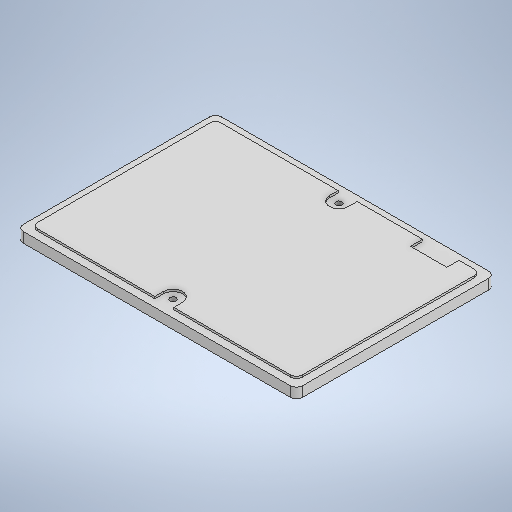
# Autodesk Inventor part: Lid
Saved by Autodesk Inventor 2025 (Build 290162000, 162)
## iProperties
Created: 2024-06-09
Part Number: Lid
Material: Generic
Document SubType Name: Modeling
Designer: Dell
Density: 1 g/cm^3
Appearance: Default
Author: Dell
Autodesk Inventor part; units mm, degrees
ref_plane "YZ Plane" through (0, 0, 0) normal (1, 0, 0) x (0, 1, 0)
ref_plane "XZ Plane" through (0, 0, 0) normal (0, 1, 0) x (-1, 0, 0)
ref_plane "XY Plane" through (0, 0, 0) normal (0, 0, 1) x (1, 0, 0)
sketch "Sketch1" plane through (0, 0, 0) normal (0, 1, 0) x (-1, 0, 0)
  line L0 (59, 49.2) -> (-66, 49.2)
  arc A0 (-66, 49.2) -> (-69, 46.2) centre (-66, 46.2) ccw
  line L1 (-69, 46.2) -> (-69, -38.8)
  arc A1 (-69, -38.8) -> (-66, -41.8) centre (-66, -38.8) ccw
  line L2 (-66, -41.8) -> (59, -41.8)
  arc A2 (59, -41.8) -> (62, -38.8) centre (59, -38.8) ccw
  line L3 (62, -38.8) -> (62, 46.2)
  arc A3 (62, 46.2) -> (59, 49.2) centre (59, 46.2) ccw
  line L4 (65.5, 49.7) -> (65.5, -42.3)
  line L5 (62.5, -45.3) -> (-69.5, -45.3)
  line L6 (-72.5, -42.3) -> (-72.5, 49.7)
  line L7 (-69.5, 52.7) -> (62.5, 52.7)
  arc A4 (62.5, -45.3) -> (65.5, -42.3) centre (62.5, -42.3) ccw
  arc A5 (-72.5, -42.3) -> (-69.5, -45.3) centre (-69.5, -42.3) ccw
  arc A6 (-69.5, 52.7) -> (-72.5, 49.7) centre (-69.5, 49.7) ccw
  arc A7 (65.5, 49.7) -> (62.5, 52.7) centre (62.5, 49.7) ccw
  point P0 (65.5, -38.8)
  point P1 (59, -45.3)
  dimension "d0" = 3
  dimension "d3" = 131
  dimension "d6" = 91
  dimension "d29" = 3.5
  dimension "d44" = 3
  dimension "d45" = 3
  dimension "d46" = 3
  dimension "d47" = 3
  constraints: 16 end point, 16 point on circle, 16 tangent, 8 centre point, 4 parallel, 3 equal radius, 2 point on line, 1 horizontal, 1 vertical
  measures "d0" radius of A3
  measures "d3" distance between parallel lines of L3 L1
  measures "d6" distance between parallel lines of L0 L2
  measures "d29" distance between parallel lines of L3 L4
  measures "d44" radius of A4
  measures "d45" radius of A5
  measures "d46" radius of A6
  measures "d47" radius of A7
extrude "Extrusion6" add sketch "Sketch1" along normal blind 1.5 contours A3 L3 A2 L2 A1 L1 A0 L0
extrude "Extrusion7" add sketch "Sketch1" along normal blind 5
sketch "Sketch3" plane through (0, 1.5, 0) normal (0, 1, 0) x (1, 0, 0)
  line L0 (-59, 41.8) -> (66, 41.8) projected
  line L1 (66, -49.2) -> (-59, -49.2) projected
  circle A0 centre (3.5, 37.3) radius 1.5
  circle A1 centre (3.5, 37.3) radius 4.5
  line L2 (8, 37.3) -> (8, 41.8)
  line L3 (-1, 37.3) -> (-1, 41.8)
  line L4 (-62, 38.8) -> (-62, -46.2) projected
  line L5 (-62, -3.7) -> (-24.2248, -3.7)
  circle A2 centre (3.5, -44.7) radius 1.5
  circle A3 centre (3.5, -44.7) radius 4.5
  line L6 (8, -44.7) -> (8, -49.2)
  line L7 (-1, -44.7) -> (-1, -49.2)
  point P0 (0, 0)
  dimension "d34" = 3
  dimension "d35" = 9
  dimension "d36" = 4.5
  constraints: 10 end point, 6 symmetric about line, 4 centre point, 4 point on circle, 2 coincident, 2 perpendicular, 2 point on line, 2 tangent, 1 horizontal, 1 midpoint, 2 other
  measures "d34" diameter of A0
  measures "d35" diameter of A1
  measures "d36" distance from line of L0 A0.centre
extrude "Extrusion8" add sketch "Sketch3" along normal blind 3.5
sketch "Sketch4" plane through (0, 1.5, 0) normal (0, 1, 0) x (1, 0, 0)
  line L0 (8, 41.8) -> (8, 37.3) projected
  arc A0 (-1, 37.3) -> (8, 37.3) centre (3.5, 37.3) ccw projected
  line L1 (-1, 37.3) -> (-1, 41.8) projected
  line L2 (-1, 41.8) -> (-59, 41.8) projected
  arc A1 (-59, 41.8) -> (-62, 38.8) centre (-59, 38.8) ccw projected
  line L3 (-62, 38.8) -> (-62, -46.2) projected
  arc A2 (-62, -46.2) -> (-59, -49.2) centre (-59, -46.2) ccw projected
  line L4 (-59, -49.2) -> (-1, -49.2) projected
  line L5 (-1, -49.2) -> (-1, -44.7) projected
  arc A3 (8, -44.7) -> (-1, -44.7) centre (3.5, -44.7) ccw projected
  line L6 (8, -44.7) -> (8, -49.2) projected
  line L7 (8, -49.2) -> (66, -49.2) projected
  arc A4 (66, -49.2) -> (69, -46.2) centre (66, -46.2) ccw projected
  line L8 (69, -46.2) -> (69, 38.8) projected
  arc A5 (69, 38.8) -> (66, 41.8) centre (66, 38.8) ccw projected
  line L9 (66, 41.8) -> (8, 41.8) projected
  line L10 (-59, 41.6) -> (-1.2, 41.6)
  line L11 (-1.2, 41.6) -> (-1.2, 37.3)
  arc A6 (-1.2, 37.3) -> (8.2, 37.3) centre (3.5, 37.3) ccw
  line L12 (8.2, 37.3) -> (8.2, 41.6)
  line L13 (8.2, 41.6) -> (66, 41.6)
  arc A7 (68.8, 38.8) -> (66, 41.6) centre (66, 38.8) ccw
  line L14 (68.8, 38.8) -> (68.8, -46.2)
  arc A8 (66, -49) -> (68.8, -46.2) centre (66, -46.2) ccw
  line L15 (66, -49) -> (8.2, -49)
  line L16 (8.2, -49) -> (8.2, -44.7)
  arc A9 (8.2, -44.7) -> (-1.2, -44.7) centre (3.5, -44.7) ccw
  line L17 (-1.2, -44.7) -> (-1.2, -49)
  line L18 (-1.2, -49) -> (-59, -49)
  arc A10 (-61.8, -46.2) -> (-59, -49) centre (-59, -46.2) ccw
  line L19 (-61.8, -46.2) -> (-61.8, 38.8)
  arc A11 (-59, 41.6) -> (-61.8, 38.8) centre (-59, 38.8) ccw
  point P0 (0, 0)
  dimension "d39" = 0.2
  constraints: 20 end point, 12 point on circle, 6 centre point, 15 other
  measures "d39" distance between parallel lines of L2 L10
extrude "Extrusion9" add sketch "Sketch4" along normal blind 3.5
extrude "Extrusion10" add sketch "Sketch4" along normal blind 4.5 contours L10 L11 A6 L12 L13 A7 L14 A8 L15 L16 A9 L17 L18 A10 L19 A11
sketch "Sketch5" plane through (0, 6, 0) normal (0, 1, 0) x (1, 0, 0)
  line L0 (66, 41.6) -> (8.2, 41.6) projected
  line L1 (40.5, 41.6) -> (58.5, 41.6)
  line L2 (58.5, 41.6) -> (58.5, 35.6)
  line L3 (58.5, 35.6) -> (40.5, 35.6)
  line L4 (40.5, 35.6) -> (40.5, 41.6)
  point P0 (0, 0)
  point P1 (69.5, 45.3)
  point P2 (49.5, 41.6)
  dimension "d48" = 18
  dimension "d49" = 6
  dimension "d50" = 20
  constraints: 8 end point, 2 parallel, 1 horizontal, 1 midpoint, 1 perpendicular, 1 point on line
  measures "d48" distance of L2.end L3.end
  measures "d49" distance of L1.end L2.end
  measures "d50" horizontal distance of point (49.5, 41.6) point (69.5, 45.3)
extrude "Extrusion11" cut sketch "Sketch5" against normal up to surface (1 mm away)
sketch "Sketch6" plane through (0, 0, 0) normal (0, -1, 0) x (1, 0, 0)
  circle A0 centre (3.5, -37.3) radius 1.5 projected
  arc A1 (8.2, -37.3) -> (-1.2, -37.3) centre (3.5, -37.3) ccw projected
  circle A2 centre (3.5, 44.7) radius 1.5 projected
  arc A3 (-1.2, 44.7) -> (8.2, 44.7) centre (3.5, 44.7) ccw projected
  circle A4 centre (3.5, -37.3) radius 2.75
  circle A5 centre (3.5, 44.7) radius 2.75
  point P0 (0, 0)
  dimension "d55" = 5.5
  dimension "d56" = 5.5
  constraints: 2 centre point, 2 coincident
  measures "d55" diameter of A4
  measures "d56" diameter of A5
extrude "Extrusion12" cut sketch "Sketch6" against normal blind 10 contours A0 | A2
extrude "Extrusion13" cut sketch "Sketch6" against normal blind 2
sketch "Sketch7" plane through (0, 0, 0) normal (0, -1, 0) x (1, 0, 0)
  line L0 (-65.5, -42.3) -> (-65.5, 49.7) projected
  line L1 (-62.5, 52.7) -> (69.5, 52.7) projected
  line L2 (72.5, 49.7) -> (72.5, -42.3) projected
  line L3 (69.5, -45.3) -> (-62.5, -45.3) projected
  line L4 (-34.3067, 8.9219) -> (41.3173, 8.9219) construction
  line L5 (41.3173, 8.9219) -> (41.3173, -1.4995) construction
  line L6 (41.3173, -1.4995) -> (-34.3067, -1.4995) construction
  line L7 (-34.3067, -1.4995) -> (-34.3067, 8.9219) construction
  line L8 (-53.3099, -3.7888) -> (-48.2532, 11.2112)
  line L9 (-48.2532, 11.2112) -> (-45.7977, 11.2112)
  line L10 (-45.7977, 11.2112) -> (-40.741, -3.7888)
  line L11 (-40.741, -3.7888) -> (-42.8439, -3.7888)
  line L12 (-42.8439, -3.7888) -> (-44.2054, 0.4049)
  line L13 (-44.2054, 0.4049) -> (-49.9306, 0.4049)
  line L14 (-49.9306, 0.4049) -> (-51.2921, -3.7888)
  line L15 (-51.2921, -3.7888) -> (-53.3099, -3.7888)
  line L16 (-44.7524, 2.1067) -> (-47.0741, 9.1691)
  line L17 (-47.0741, 9.1691) -> (-49.3836, 2.1067)
  line L18 (-49.3836, 2.1067) -> (-44.7524, 2.1067)
  spline S0 degree 2 poles (-33.0344, -4.0805) (-34.6268, -4.0805) (-37.2645, -3.1081) (-38.2127, -2.1235) knots 0 0 0 1 2 2 2
  spline S1 degree 2 poles (-38.2127, -2.1235) (-39.1608, -1.1267) (-40.1697, 1.8149) (-40.1697, 3.7234) knots 0 0 0 1 2 2 2
  spline S2 degree 2 poles (-40.1697, 3.7234) (-40.1697, 5.5346) (-39.1486, 8.4033) (-38.2005, 9.4243) knots 0 0 0 1 2 2 2
  spline S3 degree 2 poles (-38.2005, 9.4243) (-37.2888, 10.4089) (-34.6146, 11.4786) (-33.0222, 11.4786) knots 0 0 0 1 2 2 2
  spline S4 degree 2 poles (-33.0222, 11.4786) (-32.2564, 11.4786) (-30.8707, 11.2598) (-30.2386, 11.0653) knots 0 0 0 1 2 2 2
  spline S5 degree 2 poles (-30.2386, 11.0653) (-29.7281, 10.9195) (-28.4882, 10.3846) (-28.1114, 10.1901) knots 0 0 0 1 2 2 2
  line L19 (-28.1114, 10.1901) -> (-28.1114, 7.7833)
  line L20 (-28.1114, 7.7833) -> (-28.2815, 7.7833)
  spline S6 degree 2 poles (-28.2815, 7.7833) (-28.6584, 8.1115) (-29.4485, 8.7072) (-30.1778, 9.0475) knots 0 0 0 1 2 2 2
  spline S7 degree 2 poles (-30.1778, 9.0475) (-30.7856, 9.3514) (-32.3537, 9.7525) (-33.2532, 9.7525) knots 0 0 0 1 2 2 2
  spline S8 degree 2 poles (-33.2532, 9.7525) (-35.4169, 9.7525) (-38.0911, 6.4948) (-38.0911, 3.7841) knots 0 0 0 1 2 2 2
  spline S9 degree 2 poles (-38.0911, 3.7841) (-38.0911, 2.2769) (-37.3861, 0.0159) (-36.7175, -0.762) knots 0 0 0 1 2 2 2
  spline S10 degree 2 poles (-36.7175, -0.762) (-36.0733, -1.54) (-34.2499, -2.3544) (-33.1073, -2.3544) knots 0 0 0 1 2 2 2
  spline S11 degree 2 poles (-33.1073, -2.3544) (-32.2686, -2.3544) (-30.5911, -2.1113) (-30.0198, -1.8682) knots 0 0 0 1 2 2 2
  line L21 (-30.0198, -1.8682) -> (-30.0198, 2.0094)
  line L22 (-30.0198, 2.0094) -> (-33.4963, 2.0094)
  line L23 (-33.4963, 2.0094) -> (-33.4963, 3.7598)
  line L24 (-33.4963, 3.7598) -> (-28.0506, 3.7598)
  line L25 (-28.0506, 3.7598) -> (-28.0506, -2.792)
  spline S12 degree 2 poles (-28.0506, -2.792) (-28.4274, -2.9622) (-29.7159, -3.4849) (-30.2629, -3.6429) knots 0 0 0 1 2 2 2
  spline S13 degree 2 poles (-30.2629, -3.6429) (-31.0044, -3.8617) (-32.1956, -4.0805) (-33.0344, -4.0805) knots 0 0 0 1 2 2 2
  line L26 (-13.9379, -3.7888) -> (-16.5271, -3.7888)
  line L27 (-16.5271, -3.7888) -> (-21.2678, 2.1796)
  line L28 (-21.2678, 2.1796) -> (-23.553, 2.1796)
  line L29 (-23.553, 2.1796) -> (-23.553, -3.7888)
  line L30 (-23.553, -3.7888) -> (-25.5465, -3.7888)
  line L31 (-25.5465, -3.7888) -> (-25.5465, 11.2112)
  line L32 (-25.5465, 11.2112) -> (-21.681, 11.2112)
  spline S14 degree 2 poles (-21.681, 11.2112) (-20.3926, 11.2112) (-18.6543, 10.9316) (-17.8642, 10.4211) knots 0 0 0 1 2 2 2
  spline S15 degree 2 poles (-17.8642, 10.4211) (-17.0741, 9.9106) (-16.1624, 8.3182) (-16.1624, 7.1391) knots 0 0 0 1 2 2 2
  spline S16 degree 2 poles (-16.1624, 7.1391) (-16.1624, 5.4981) (-17.8399, 3.2736) (-19.2742, 2.7388) knots 0 0 0 1 2 2 2
  line L33 (-19.2742, 2.7388) -> (-13.9379, -3.7888)
  spline S17 degree 2 poles (-18.241, 6.9811) (-18.241, 7.6375) (-18.7029, 8.6464) (-19.1892, 8.9746) knots 0 0 0 1 2 2 2
  spline S18 degree 2 poles (-19.1892, 8.9746) (-19.6146, 9.2542) (-20.7451, 9.4851) (-21.5716, 9.4851) knots 0 0 0 1 2 2 2
  line L34 (-21.5716, 9.4851) -> (-23.553, 9.4851)
  line L35 (-23.553, 9.4851) -> (-23.553, 3.8449)
  line L36 (-23.553, 3.8449) -> (-21.8026, 3.8449)
  spline S19 degree 2 poles (-21.8026, 3.8449) (-20.9396, 3.8449) (-19.566, 4.1488) (-19.0919, 4.6229) knots 0 0 0 1 2 2 2
  spline S20 degree 2 poles (-19.0919, 4.6229) (-18.6543, 5.0362) (-18.241, 6.2031) (-18.241, 6.9811) knots 0 0 0 1 2 2 2
  spline S21 degree 2 poles (-2.1349, 9.4973) (-1.284, 8.5005) (-0.3358, 5.5832) (-0.3358, 3.7112) knots 0 0 0 1 2 2 2
  spline S22 degree 2 poles (-0.3358, 3.7112) (-0.3358, 1.8879) (-1.2597, -1.0659) (-2.1349, -2.0627) knots 0 0 0 1 2 2 2
  spline S23 degree 2 poles (-2.1349, -2.0627) (-3.0587, -3.1081) (-5.502, -4.1048) (-6.9728, -4.1048) knots 0 0 0 1 2 2 2
  spline S24 degree 2 poles (-6.9728, -4.1048) (-8.4922, -4.1048) (-10.9234, -3.0716) (-11.8107, -2.0627) knots 0 0 0 1 2 2 2
  spline S25 degree 2 poles (-11.8107, -2.0627) (-12.6738, -1.0659) (-13.5976, 1.8636) (-13.5976, 3.7112) knots 0 0 0 1 2 2 2
  spline S26 degree 2 poles (-13.5976, 3.7112) (-13.5976, 5.5953) (-12.6616, 8.4641) (-11.7986, 9.4973) knots 0 0 0 1 2 2 2
  spline S27 degree 2 poles (-11.7986, 9.4973) (-10.9234, 10.494) (-8.4801, 11.5273) (-6.9728, 11.5273) knots 0 0 0 1 2 2 2
  spline S28 degree 2 poles (-6.9728, 11.5273) (-5.4412, 11.5273) (-2.9857, 10.4576) (-2.1349, 9.4973) knots 0 0 0 1 2 2 2
  spline S29 degree 2 poles (-2.4144, 3.7112) (-2.4144, 5.1942) (-3.0587, 7.4916) (-3.6422, 8.2452) knots 0 0 0 1 2 2 2
  spline S30 degree 2 poles (-3.6422, 8.2452) (-4.2378, 9.0232) (-5.9152, 9.8012) (-6.9606, 9.8012) knots 0 0 0 1 2 2 2
  spline S31 degree 2 poles (-6.9606, 9.8012) (-8.0425, 9.8012) (-9.6713, 9.0475) (-10.2913, 8.2452) knots 0 0 0 1 2 2 2
  spline S32 degree 2 poles (-10.2913, 8.2452) (-10.8869, 7.4794) (-11.519, 5.1699) (-11.519, 3.7112) knots 0 0 0 1 2 2 2
  spline S33 degree 2 poles (-11.519, 3.7112) (-11.519, 0.7574) (-9.0392, -2.3787) (-6.9606, -2.3787) knots 0 0 0 1 2 2 2
  spline S34 degree 2 poles (-6.9606, -2.3787) (-4.882, -2.3787) (-2.4144, 0.7574) (-2.4144, 3.7112) knots 0 0 0 1 2 2 2
  spline S35 degree 2 poles (6.0337, -4.0562) (4.4049, -4.0562) (2.1196, -3.3755) (1.1107, -2.8893) knots 0 0 0 1 2 2 2
  line L37 (1.1107, -2.8893) -> (1.1107, -0.3852)
  line L38 (1.1107, -0.3852) -> (1.2566, -0.3852)
  spline S36 degree 2 poles (1.2566, -0.3852) (2.2412, -1.309) (4.7331, -2.3301) (5.8878, -2.3301) knots 0 0 0 1 2 2 2
  spline S37 degree 2 poles (5.8878, -2.3301) (7.541, -2.3301) (9.2306, -0.9565) (9.2306, 0.1739) knots 0 0 0 1 2 2 2
  spline S38 degree 2 poles (9.2306, 0.1739) (9.2306, 1.0735) (8.3433, 2.1918) (7.383, 2.4713) knots 0 0 0 1 2 2 2
  spline S39 degree 2 poles (7.383, 2.4713) (6.6901, 2.6658) (5.5353, 2.9333) (4.6723, 3.1521) knots 0 0 0 1 2 2 2
  spline S40 degree 2 poles (4.6723, 3.1521) (3.8943, 3.3587) (2.6666, 3.9786) (2.1925, 4.477) knots 0 0 0 1 2 2 2
  spline S41 degree 2 poles (2.1925, 4.477) (1.7306, 4.9754) (1.2201, 6.3125) (1.2201, 7.1877) knots 0 0 0 1 2 2 2
  spline S42 degree 2 poles (1.2201, 7.1877) (1.2201, 9.0111) (4.0645, 11.4786) (6.2647, 11.4786) knots 0 0 0 1 2 2 2
  spline S43 degree 2 poles (6.2647, 11.4786) (7.5288, 11.4786) (9.7655, 10.9803) (10.7258, 10.5062) knots 0 0 0 1 2 2 2
  line L39 (10.7258, 10.5062) -> (10.7258, 8.1237)
  line L40 (10.7258, 8.1237) -> (10.5799, 8.1237)
  spline S44 degree 2 poles (10.5799, 8.1237) (9.8627, 8.7801) (7.6261, 9.7525) (6.3984, 9.7525) knots 0 0 0 1 2 2 2
  spline S45 degree 2 poles (6.3984, 9.7525) (5.0126, 9.7525) (3.2987, 8.4519) (3.2987, 7.3944) knots 0 0 0 1 2 2 2
  spline S46 degree 2 poles (3.2987, 7.3944) (3.2987, 6.4462) (4.3076, 5.3158) (5.2557, 5.0605) knots 0 0 0 1 2 2 2
  spline S47 degree 2 poles (5.2557, 5.0605) (5.8878, 4.8903) (7.7233, 4.4527) (8.3311, 4.2704) knots 0 0 0 1 2 2 2
  spline S48 degree 2 poles (8.3311, 4.2704) (9.8749, 3.7963) (11.3092, 1.8879) (11.3092, 0.49) knots 0 0 0 1 2 2 2
  spline S49 degree 2 poles (11.3092, 0.49) (11.3092, -0.3974) (10.592, -2.0992) (9.9478, -2.6948) knots 0 0 0 1 2 2 2
  spline S50 degree 2 poles (9.9478, -2.6948) (9.2306, -3.3512) (7.4073, -4.0562) (6.0337, -4.0562) knots 0 0 0 1 2 2 2
  line L41 (13.3392, -3.7888) -> (13.3392, 11.2112)
  line L42 (13.3392, 11.2112) -> (22.7233, 11.2112)
  line L43 (22.7233, 11.2112) -> (22.7233, 9.4365)
  line L44 (22.7233, 9.4365) -> (15.3327, 9.4365)
  line L45 (15.3327, 9.4365) -> (15.3327, 5.3279)
  line L46 (15.3327, 5.3279) -> (22.2249, 5.3279)
  line L47 (22.2249, 5.3279) -> (22.2249, 3.5532)
  line L48 (22.2249, 3.5532) -> (15.3327, 3.5532)
  line L49 (15.3327, 3.5532) -> (15.3327, -2.0141)
  line L50 (15.3327, -2.0141) -> (22.7233, -2.0141)
  line L51 (22.7233, -2.0141) -> (22.7233, -3.7888)
  line L52 (22.7233, -3.7888) -> (13.3392, -3.7888)
  line L53 (35.6447, -3.7888) -> (33.4081, -3.7888)
  line L54 (33.4081, -3.7888) -> (26.7711, 9.1448)
  line L55 (26.7711, 9.1448) -> (26.7711, -3.7888)
  line L56 (26.7711, -3.7888) -> (24.9113, -3.7888)
  line L57 (24.9113, -3.7888) -> (24.9113, 11.2112)
  line L58 (24.9113, 11.2112) -> (27.7436, 11.2112)
  line L59 (27.7436, 11.2112) -> (33.7849, -0.6648)
  line L60 (33.7849, -0.6648) -> (33.7849, 11.2112)
  line L61 (33.7849, 11.2112) -> (35.6447, 11.2112)
  line L62 (35.6447, 11.2112) -> (35.6447, -3.7888)
  spline S51 degree 2 poles (42.8651, -4.0562) (41.2363, -4.0562) (38.951, -3.3755) (37.9421, -2.8893) knots 0 0 0 1 2 2 2
  line L63 (37.9421, -2.8893) -> (37.9421, -0.3852)
  line L64 (37.9421, -0.3852) -> (38.088, -0.3852)
  spline S52 degree 2 poles (38.088, -0.3852) (39.0726, -1.309) (41.5645, -2.3301) (42.7193, -2.3301) knots 0 0 0 1 2 2 2
  spline S53 degree 2 poles (42.7193, -2.3301) (44.3724, -2.3301) (46.0621, -0.9565) (46.0621, 0.1739) knots 0 0 0 1 2 2 2
  spline S54 degree 2 poles (46.0621, 0.1739) (46.0621, 1.0735) (45.1747, 2.1918) (44.2144, 2.4713) knots 0 0 0 1 2 2 2
  spline S55 degree 2 poles (44.2144, 2.4713) (43.5215, 2.6658) (42.3668, 2.9333) (41.5037, 3.1521) knots 0 0 0 1 2 2 2
  spline S56 degree 2 poles (41.5037, 3.1521) (40.7258, 3.3587) (39.498, 3.9786) (39.024, 4.477) knots 0 0 0 1 2 2 2
  spline S57 degree 2 poles (39.024, 4.477) (38.5621, 4.9754) (38.0515, 6.3125) (38.0515, 7.1877) knots 0 0 0 1 2 2 2
  spline S58 degree 2 poles (38.0515, 7.1877) (38.0515, 9.0111) (40.8959, 11.4786) (43.0961, 11.4786) knots 0 0 0 1 2 2 2
  spline S59 degree 2 poles (43.0961, 11.4786) (44.3603, 11.4786) (46.5969, 10.9803) (47.5572, 10.5062) knots 0 0 0 1 2 2 2
  line L65 (47.5572, 10.5062) -> (47.5572, 8.1237)
  line L66 (47.5572, 8.1237) -> (47.4113, 8.1237)
  spline S60 degree 2 poles (47.4113, 8.1237) (46.6942, 8.7801) (44.4575, 9.7525) (43.2298, 9.7525) knots 0 0 0 1 2 2 2
  spline S61 degree 2 poles (43.2298, 9.7525) (41.8441, 9.7525) (40.1301, 8.4519) (40.1301, 7.3944) knots 0 0 0 1 2 2 2
  spline S62 degree 2 poles (40.1301, 7.3944) (40.1301, 6.4462) (41.139, 5.3158) (42.0872, 5.0605) knots 0 0 0 1 2 2 2
  spline S63 degree 2 poles (42.0872, 5.0605) (42.7193, 4.8903) (44.5548, 4.4527) (45.1625, 4.2704) knots 0 0 0 1 2 2 2
  spline S64 degree 2 poles (45.1625, 4.2704) (46.7063, 3.7963) (48.1407, 1.8879) (48.1407, 0.49) knots 0 0 0 1 2 2 2
  spline S65 degree 2 poles (48.1407, 0.49) (48.1407, -0.3974) (47.4235, -2.0992) (46.7792, -2.6948) knots 0 0 0 1 2 2 2
  spline S66 degree 2 poles (46.7792, -2.6948) (46.0621, -3.3512) (44.2387, -4.0562) (42.8651, -4.0562) knots 0 0 0 1 2 2 2
  line L67 (50.1707, -3.7888) -> (50.1707, 11.2112)
  line L68 (50.1707, 11.2112) -> (59.5548, 11.2112)
  line L69 (59.5548, 11.2112) -> (59.5548, 9.4365)
  line L70 (59.5548, 9.4365) -> (52.1642, 9.4365)
  line L71 (52.1642, 9.4365) -> (52.1642, 5.3279)
  line L72 (52.1642, 5.3279) -> (59.0564, 5.3279)
  line L73 (59.0564, 5.3279) -> (59.0564, 3.5532)
  line L74 (59.0564, 3.5532) -> (52.1642, 3.5532)
  line L75 (52.1642, 3.5532) -> (52.1642, -2.0141)
  line L76 (52.1642, -2.0141) -> (59.5548, -2.0141)
  line L77 (59.5548, -2.0141) -> (59.5548, -3.7888)
  line L78 (59.5548, -3.7888) -> (50.1707, -3.7888)
  point P0 (0, 0)
  point P1 (3.5, 52.7)
  point P2 (-65.5, 3.7)
  point P3 (3.5, 3.7)
  constraints: 2 midpoint, 2 other
extrude "Extrusion15" cut sketch "Sketch7" against normal blind 1
body "Solid3"
